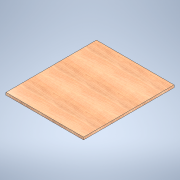
# Autodesk Inventor part: basePlate
Saved by Autodesk Inventor 2022.2 (Build 262287000, 287)
## iProperties
Created: 2022-01-19
Part Number: basePlate
Material: Wood (Birch)
Document SubType Name: Modeling
Designer: robst
Density: 0.55 g/cm^3
Appearance: Birch - Natural Polished
Author: robst
Autodesk Inventor part; units mm, degrees
ref_plane "YZ Plane" through (0, 0, 0) normal (1, 0, 0) x (0, 1, 0)
ref_plane "XZ Plane" through (0, 0, 0) normal (0, 1, 0) x (-1, 0, 0)
ref_plane "XY Plane" through (0, 0, 0) normal (0, 0, 1) x (1, 0, 0)
sketch "Sketch1" plane through (0, 0, 0) normal (0, 1, 0) x (-1, 0, 0)
  line L0 (304.8, 355.6) -> (-304.8, 355.6)
  line L1 (-304.8, 355.6) -> (-304.8, -355.6)
  line L2 (-304.8, -355.6) -> (304.8, -355.6)
  line L3 (304.8, -355.6) -> (304.8, 355.6)
  line L4 (304.8, 355.6) -> (-304.8, -355.6) construction
  line L5 (-304.8, 355.6) -> (304.8, -355.6) construction
  point P0 (0, 0)
  dimension "d0" = 609.6
  dimension "d1" = 711.2
  constraints: 12 end point, 2 midpoint, 2 parallel, 1 horizontal, 1 perpendicular
  measures "d0" distance of L0.start L0.end
  measures "d1" distance of L1.end L0.end
extrude "Extrusion1" add sketch "Sketch1" against normal blind 19.05
body "Solid1"
